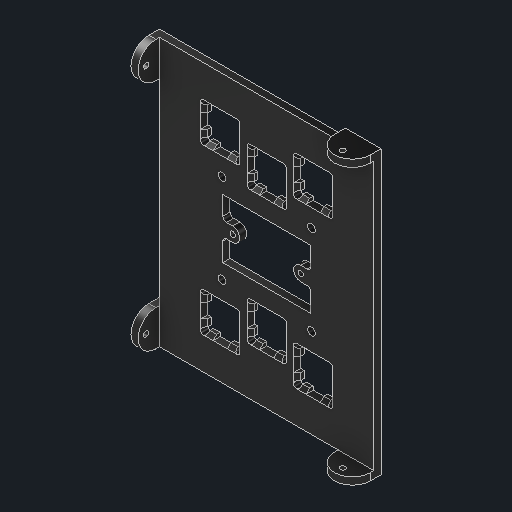
# Autodesk Inventor part: LED_mount
Saved by Autodesk Inventor 2026.1 (Build 301233000, 233)
## iProperties
Created: 2026-01-20
Part Number: LED_mount
Material: ABS Plastic
Document SubType Name: Modeling
Designer: aleja
Density: 1.06 g/cm^3
Appearance: Glossy - Black
Author: aleja
Autodesk Inventor part; units mm, degrees
ref_plane "YZ Plane" through (0, 0, 0) normal (1, 0, 0) x (0, 1, 0)
ref_plane "XZ Plane" through (0, 0, 0) normal (0, 1, 0) x (-1, 0, 0)
ref_plane "XY Plane" through (0, 0, 0) normal (0, 0, 1) x (1, 0, 0)
sketch "Sketch1" plane through (0, 0, 0) normal (0, 1, 0) x (-1, 0, 0)
  line L0 (-60, 75) -> (60, 75)
  line L1 (60, 75) -> (60, -75)
  line L2 (60, -75) -> (-60, -75)
  line L3 (-60, -75) -> (-60, 75)
  line L4 (-60, 75) -> (60, -75) construction
  line L5 (60, 75) -> (-60, -75) construction
  point P0 (0, 0)
  dimension "d0" = 120
  dimension "d1" = 150
  constraints: 12 end point, 2 midpoint, 2 parallel, 1 horizontal, 1 perpendicular
  measures "d0" distance of L1.end L2.end
  measures "d1" distance of L0.end L1.end
extrude "Extrusion1" add sketch "Sketch1" along normal blind 4
sketch "Sketch3" plane through (0, 0, 0) normal (0, -1, 0) x (1, 0, 0)
  line L0 (-60, 75) -> (60, 75) projected
  line L1 (-60, 75) -> (-64, 75)
  line L2 (-64, 75) -> (-64, 55)
  line L3 (-64, 55) -> (-60, 55)
  line L4 (-60, 55) -> (-60, 75)
  line L5 (-64, 75) -> (-40, 75)
  line L6 (-40, 75) -> (-40, 79)
  line L7 (-40, 79) -> (-64, 79)
  line L8 (-64, 79) -> (-64, 75)
  line L9 (-60, -75) -> (-60, 75) projected
  line L10 (-60, 0) -> (-43.5069, 0) construction
  line L11 (-60, -75) -> (-64, -75)
  line L12 (-64, -75) -> (-64, -55)
  line L13 (-64, -55) -> (-60, -55)
  line L14 (-60, -55) -> (-60, -75)
  line L15 (-64, -75) -> (-40, -75)
  line L16 (-40, -75) -> (-40, -79)
  line L17 (-40, -79) -> (-64, -79)
  line L18 (-64, -79) -> (-64, -75)
  line L19 (0, 75) -> (0, 63.1817) construction
  line L20 (60, 75) -> (64, 75)
  line L21 (64, 75) -> (64, 55)
  line L22 (64, 55) -> (60, 55)
  line L23 (60, 55) -> (60, 75)
  line L24 (64, 75) -> (40, 75)
  line L25 (40, 75) -> (40, 79)
  line L26 (40, 79) -> (64, 79)
  line L27 (64, 79) -> (64, 75)
  line L28 (60, -75) -> (60, 75)
  line L29 (60, 0) -> (43.5069, 0) construction
  line L30 (60, -75) -> (64, -75)
  line L31 (64, -75) -> (64, -55)
  line L32 (64, -55) -> (60, -55)
  line L33 (60, -55) -> (60, -75)
  line L34 (64, -75) -> (40, -75)
  line L35 (40, -75) -> (40, -79)
  line L36 (40, -79) -> (64, -79)
  line L37 (64, -79) -> (64, -75)
  line L38 (60, -75) -> (60, -79)
  line L39 (60, 75) -> (60, 79)
  point P0 (0, 0)
  dimension "d21" = 4
  dimension "d22" = 20
  dimension "d23" = 24
  dimension "d24" = 4
  constraints: 76 end point, 21 symmetric about line, 4 parallel, 3 horizontal, 3 perpendicular, 3 point on line, 2 midpoint, 1 vertical
  measures "d21" distance of L3.end L2.end
  measures "d22" distance of L2.end L1.end
  measures "d23" distance of L7.end L6.end
  measures "d24" distance of L6.end L5.end
extrude "Extrusion3" add sketch "Sketch3" along normal blind 15 and the other way blind 4 contours L4 L3 L2 L1 | L25 L26 L39 L0 | L11 L12 L13 L9 | L38 L36 L35 L34
sketch "Sketch2" plane through (0, 0, 0) normal (0, 1, 0) x (1, 0, 0)
  line L0 (24.55, -16.5) -> (-24.55, -16.5)
  line L1 (-24.55, -16.5) -> (-24.55, 16.5)
  line L2 (-24.55, 16.5) -> (24.55, 16.5)
  line L3 (24.55, 16.5) -> (24.55, -16.5)
  line L4 (24.55, -16.5) -> (-24.55, 16.5) construction
  line L5 (-24.55, -16.5) -> (24.55, 16.5) construction
  line L6 (-24.55, 0) -> (-19.05, 0) construction
  line L7 (0, 0) -> (0, 7.7901) construction
  line L8 (37, -57) -> (15, -57) construction
  line L9 (15, -57) -> (15, -35) construction
  line L10 (15, -35) -> (37, -35) construction
  line L11 (37, -35) -> (37, -57) construction
  line L12 (0, 0) -> (-54.7536, 0) construction
  line L13 (0, 0) -> (0, -64.3839) construction
  line L14 (-24.55, -4) -> (-19.05, -4)
  arc A0 (-19.05, -4) -> (-19.05, 4) centre (-19.05, 0) ccw
  line L15 (-24.55, 4) -> (-19.05, 4)
  circle A1 centre (-19.05, 0) radius 1.5
  line L16 (24.55, -4) -> (19.05, -4)
  arc A2 (19.05, 4) -> (19.05, -4) centre (19.05, 0) ccw
  line L17 (24.55, 4) -> (19.05, 4)
  circle A3 centre (19.05, 0) radius 1.5
  line L18 (35.4, -36.6) -> (16.6, -36.6) construction
  line L19 (16.6, -36.6) -> (16.6, -55.4) construction
  line L20 (16.6, -55.4) -> (35.4, -55.4) construction
  line L21 (35.4, -55.4) -> (35.4, -36.6) construction
  arc A4 (35, -38.1492) -> (33.8508, -37) centre (35.4, -36.6) ccw
  line L22 (26, -36.6) -> (26, -55.4) construction
  line L23 (35.4, -46) -> (16.6, -46) construction
  arc A5 (18.1492, -37) -> (17, -38.1492) centre (16.6, -36.6) ccw
  arc A6 (33.8508, -55) -> (35, -53.8508) centre (35.4, -55.4) ccw
  arc A7 (17, -53.8508) -> (18.1492, -55) centre (16.6, -55.4) ccw
  line L24 (33.8508, -37) -> (18.1492, -37)
  line L25 (33.8508, -55) -> (18.1492, -55)
  line L26 (35.4, -36.6) -> (16.6, -55.4) construction
  line L27 (16.6, -36.6) -> (35.4, -55.4) construction
  line L28 (17, -53.8508) -> (17, -38.1492)
  line L29 (35, -53.8508) -> (35, -38.1492)
  line L30 (11, -48.5) -> (-11, -48.5) construction
  line L31 (-11, -48.5) -> (-11, -26.5) construction
  line L32 (-11, -26.5) -> (11, -26.5) construction
  line L33 (11, -26.5) -> (11, -48.5) construction
  line L34 (9.4, -28.1) -> (-9.4, -28.1) construction
  line L35 (-9.4, -28.1) -> (-9.4, -46.9) construction
  line L36 (-9.4, -46.9) -> (9.4, -46.9) construction
  line L37 (9.4, -46.9) -> (9.4, -28.1) construction
  arc A8 (9, -29.6492) -> (7.8508, -28.5) centre (9.4, -28.1) ccw
  line L38 (0, -28.1) -> (0, -46.9) construction
  line L39 (9.4, -37.5) -> (-9.4, -37.5) construction
  arc A9 (-7.8508, -28.5) -> (-9, -29.6492) centre (-9.4, -28.1) ccw
  arc A10 (7.8508, -46.5) -> (9, -45.3508) centre (9.4, -46.9) ccw
  arc A11 (-9, -45.3508) -> (-7.8508, -46.5) centre (-9.4, -46.9) ccw
  line L40 (7.8508, -28.5) -> (-7.8508, -28.5)
  line L41 (7.8508, -46.5) -> (-7.8508, -46.5)
  line L42 (9.4, -28.1) -> (-9.4, -46.9) construction
  line L43 (-9.4, -28.1) -> (9.4, -46.9) construction
  line L44 (-9, -45.3508) -> (-9, -29.6492)
  line L45 (9, -45.3508) -> (9, -29.6492)
  line L46 (-37, -57) -> (-15, -57) construction
  line L47 (-15, -57) -> (-15, -35) construction
  line L48 (-15, -35) -> (-37, -35) construction
  line L49 (-37, -35) -> (-37, -57) construction
  line L50 (-35.4, -36.6) -> (-16.6, -36.6) construction
  line L51 (-16.6, -36.6) -> (-16.6, -55.4) construction
  line L52 (-16.6, -55.4) -> (-35.4, -55.4) construction
  line L53 (-35.4, -55.4) -> (-35.4, -36.6) construction
  arc A12 (-33.8508, -37) -> (-35, -38.1492) centre (-35.4, -36.6) ccw
  line L54 (-26, -36.6) -> (-26, -55.4) construction
  line L55 (-35.4, -46) -> (-16.6, -46) construction
  arc A13 (-17, -38.1492) -> (-18.1492, -37) centre (-16.6, -36.6) ccw
  arc A14 (-35, -53.8508) -> (-33.8508, -55) centre (-35.4, -55.4) ccw
  arc A15 (-18.1492, -55) -> (-17, -53.8508) centre (-16.6, -55.4) ccw
  line L56 (-33.8508, -37) -> (-18.1492, -37)
  line L57 (-33.8508, -55) -> (-18.1492, -55)
  line L58 (-35.4, -36.6) -> (-16.6, -55.4) construction
  line L59 (-16.6, -36.6) -> (-35.4, -55.4) construction
  line L60 (-17, -53.8508) -> (-17, -38.1492)
  line L61 (-35, -53.8508) -> (-35, -38.1492)
  line L62 (37, 57) -> (15, 57) construction
  line L63 (15, 57) -> (15, 35) construction
  line L64 (15, 35) -> (37, 35) construction
  line L65 (37, 35) -> (37, 57) construction
  line L66 (0, 0) -> (0, 64.3839) construction
  line L67 (35.4, 36.6) -> (16.6, 36.6) construction
  line L68 (16.6, 36.6) -> (16.6, 55.4) construction
  line L69 (16.6, 55.4) -> (35.4, 55.4) construction
  line L70 (35.4, 55.4) -> (35.4, 36.6) construction
  arc A16 (33.8508, 37) -> (35, 38.1492) centre (35.4, 36.6) ccw
  line L71 (26, 36.6) -> (26, 55.4) construction
  line L72 (35.4, 46) -> (16.6, 46) construction
  arc A17 (17, 38.1492) -> (18.1492, 37) centre (16.6, 36.6) ccw
  arc A18 (35, 53.8508) -> (33.8508, 55) centre (35.4, 55.4) ccw
  arc A19 (18.1492, 55) -> (17, 53.8508) centre (16.6, 55.4) ccw
  line L73 (33.8508, 37) -> (18.1492, 37)
  line L74 (33.8508, 55) -> (18.1492, 55)
  line L75 (35.4, 36.6) -> (16.6, 55.4) construction
  line L76 (16.6, 36.6) -> (35.4, 55.4) construction
  line L77 (17, 53.8508) -> (17, 38.1492)
  line L78 (35, 53.8508) -> (35, 38.1492)
  arc A20 (7.8508, 28.5) -> (9, 29.6492) centre (9.4, 28.1) ccw
  line L79 (9, 45.3508) -> (9, 29.6492)
  line L80 (9.4, 46.9) -> (9.4, 28.1) construction
  line L81 (11, 26.5) -> (11, 48.5) construction
  arc A21 (9, 45.3508) -> (7.8508, 46.5) centre (9.4, 46.9) ccw
  line L82 (7.8508, 28.5) -> (-7.8508, 28.5)
  line L83 (-11, 26.5) -> (11, 26.5) construction
  line L84 (0, 28.1) -> (0, 46.9) construction
  line L85 (9.4, 28.1) -> (-9.4, 28.1) construction
  line L86 (9.4, 37.5) -> (-9.4, 37.5) construction
  line L87 (-9, 45.3508) -> (-9, 29.6492)
  line L88 (-9.4, 28.1) -> (9.4, 46.9) construction
  line L89 (9.4, 28.1) -> (-9.4, 46.9) construction
  line L90 (-9.4, 28.1) -> (-9.4, 46.9) construction
  line L91 (7.8508, 46.5) -> (-7.8508, 46.5)
  line L92 (-9.4, 46.9) -> (9.4, 46.9) construction
  line L93 (11, 48.5) -> (-11, 48.5) construction
  line L94 (-11, 48.5) -> (-11, 26.5) construction
  arc A22 (-9, 29.6492) -> (-7.8508, 28.5) centre (-9.4, 28.1) ccw
  arc A23 (-7.8508, 46.5) -> (-9, 45.3508) centre (-9.4, 46.9) ccw
  line L95 (-37, 57) -> (-15, 57) construction
  line L96 (-15, 57) -> (-15, 35) construction
  line L97 (-33.8508, 55) -> (-18.1492, 55)
  line L98 (-16.6, 36.6) -> (-35.4, 55.4) construction
  line L99 (-35.4, 36.6) -> (-16.6, 55.4) construction
  arc A24 (-17, 53.8508) -> (-18.1492, 55) centre (-16.6, 55.4) ccw
  line L100 (-16.6, 55.4) -> (-35.4, 55.4) construction
  line L101 (-16.6, 36.6) -> (-16.6, 55.4) construction
  line L102 (-17, 53.8508) -> (-17, 38.1492)
  line L103 (-35.4, 46) -> (-16.6, 46) construction
  line L104 (-33.8508, 37) -> (-18.1492, 37)
  line L105 (-35.4, 36.6) -> (-16.6, 36.6) construction
  arc A25 (-18.1492, 37) -> (-17, 38.1492) centre (-16.6, 36.6) ccw
  line L106 (-15, 35) -> (-37, 35) construction
  arc A26 (-35, 38.1492) -> (-33.8508, 37) centre (-35.4, 36.6) ccw
  line L107 (-26, 36.6) -> (-26, 55.4) construction
  line L108 (-35, 53.8508) -> (-35, 38.1492)
  line L109 (-37, 35) -> (-37, 57) construction
  arc A27 (-33.8508, 55) -> (-35, 53.8508) centre (-35.4, 55.4) ccw
  line L110 (-35.4, 55.4) -> (-35.4, 36.6) construction
  point P0 (19.05, 0)
  dimension "d4" = 49.1
  dimension "d5" = 33
  dimension "d64" = 22
  dimension "d66" = 15
  dimension "d68" = 35
  dimension "d82" = 5.5
  dimension "d83" = 3
  dimension "d85" = 8
  dimension "d119" = 18.8
  dimension "d120" = 3.2
  dimension "d121" = 2
  dimension "d122" = 22
  dimension "d123" = 18.8
  dimension "d124" = 3.2
  dimension "d125" = 2
  dimension "d126" = 10
  constraints: 222 end point, 122 symmetric about line, 52 point on circle, 28 centre point, 11 midpoint, 10 parallel, 9 horizontal, 8 coincident, 7 perpendicular, 4 tangent, 3 point on line, 2 vertical, 1 collinear, 30 other
  measures "d4" distance of L1.end L2.end
  measures "d5" distance of L0.end L1.end
  measures "d64" distance of L8.start L8.end
  measures "d66" distance from line of L7.start L9
  measures "d68" distance from line of L7.start L10
  measures "d82" distance of L15.end L15.start
  measures "d83" diameter of A1
  measures "d85" distance between parallel lines of L15 L14
  measures "d119" distance of L20.end L18.start
  measures "d120" diameter of A4
  measures "d121" distance between parallel lines of L10 L24
  measures "d122" distance of L33.end L30.end
  measures "d123" distance of L37.start L37.end
  measures "d124" diameter of A8
  measures "d125" distance between parallel lines of L32 L40
  measures "d126" distance between parallel lines of L0 L32
extrude "Extrusion2" cut sketch "Sketch2" along normal through all contours L0 L1 L14 A0 L15 L2 L3 L17 A2 L16 | A1 | A3 | L29 A6 L25 A7 L28 A5 L24 A4 | L45 A10 L41 A11 L44 A9 L40 A8 | L56 A13 L60 A15 L57 A14 L61 A12 | L73 A17 L77 A19 L74 A18 L78 A16 | L82 A22 L87 A23 L91 A21 L79 A20 | L97 A24 L102 A25 L104 A26 L108 A27
sketch "Sketch7" plane through (-60, 0, -55) normal (1, 0, 0) x (0, 0, -1)
  line L0 (0, -15) -> (20, -15) projected
  line L1 (10, -15) -> (10, 0)
  line L2 (20, 0) -> (0, 0) projected
  circle A0 centre (10, -7.5) radius 1.5
  line L3 (-55, 0) -> (-55, -12.3055)
  circle A1 centre (-120, -7.5) radius 1.5
  dimension "d47" = 3
  constraints: 4 end point, 3 midpoint, 2 centre point, 1 symmetric about line, 1 vertical, 1 other
  measures "d47" diameter of A0
extrude "Extrusion8" cut sketch "Sketch7" against normal through all
sketch "Sketch8" plane through (60, 0, 75) normal (0, 0, -1) x (-1, 0, 0)
  line L0 (20, -15) -> (0, -15) projected
  line L1 (10, -15) -> (10, 0)
  line L2 (20, 0) -> (0, 0) projected
  circle A0 centre (10, -7.5) radius 1.5
  point P0 (60, 0)
  dimension "d50" = 3
  constraints: 3 midpoint, 2 end point, 1 centre point
  measures "d50" diameter of A0
extrude "Extrusion9" cut sketch "Sketch8" along normal through all both and the other way through all
sketch "Sketch9" plane through (0, -15, 0) normal (0, -1, 0) x (1, 0, 0)
  line L0 (-64, -55) -> (-64, -75) projected
  line L1 (-60, -75) -> (-60, -55) projected
  line L2 (-60, -55) -> (-64, -55) projected
  line L3 (-64, -75) -> (-60, -75) projected
  line L4 (-64, 55) -> (-60, 55) projected
  line L5 (-60, 55) -> (-60, 75) projected
  line L6 (-60, 75) -> (-64, 75) projected
  line L7 (-64, 75) -> (-64, 55) projected
  line L8 (60, 79) -> (40, 79) projected
  line L9 (40, 79) -> (40, 75) projected
  line L10 (40, 75) -> (60, 75) projected
  line L11 (60, 75) -> (60, 79) projected
  line L12 (40, -79) -> (60, -79) projected
  line L13 (60, -79) -> (60, -75) projected
  line L14 (60, -75) -> (40, -75) projected
  line L15 (40, -75) -> (40, -79) projected
  point P0 (0, 0)
extrude "Extrusion10" cut sketch "Sketch9" against normal blind 3
fillet "Fillet2" radius 10 8 edges at (-62, -12, -55) (-62, -12, -75) (-62, -12, 55) (-62, -12, 75) (40, -12, 77) (60, -12, 77) (60, -12, -77) (40, -12, -77)
sketch "Sketch10" plane through (0, 4, 0) normal (0, 1, 0) x (1, 0, 0)
  line L0 (25, 25) -> (-25, 25) construction
  line L1 (-25, 25) -> (-25, -25) construction
  line L2 (-25, -25) -> (25, -25) construction
  line L3 (25, -25) -> (25, 25) construction
  line L4 (25, 25) -> (-25, -25) construction
  line L5 (-25, 25) -> (25, -25) construction
  circle A0 centre (25, -25) radius 2.15
  circle A1 centre (-25, -25) radius 2.15
  circle A2 centre (-25, 25) radius 2.15
  circle A3 centre (25, 25) radius 2.15
  point P0 (0, 0)
  dimension "d56" = 50
  dimension "d57" = 50
  dimension "d58" = 4.3
  dimension "d59" = 4.3
  dimension "d60" = 4.3
  dimension "d61" = 4.3
  constraints: 12 end point, 4 centre point, 4 coincident, 2 midpoint, 2 parallel, 1 horizontal, 1 perpendicular
  measures "d56" distance of L1.end L2.end
  measures "d57" distance of L0.end L1.end
  measures "d58" diameter of A0
  measures "d59" diameter of A1
  measures "d60" diameter of A2
  measures "d61" diameter of A3
extrude "Extrusion12" cut sketch "Sketch10" against normal through all
fillet "Fillet3" radius 2 4 edges at (-24.55, 2, -4) (-24.55, 2, 4) (24.55, 2, 4) (24.55, 2, -4)
chamfer "Chamfer2" distance 2 angle 45 24 edges at (0, 0, -46.5) (26, 0, -55) (35, 0, -46) (17, 0, -46) (26, 0, -37) (9, 0, -37.5) (0, 0, -28.5) (-9, 0, -37.5) (-17, 0, -46) (-26, 0, -55) (-26, 0, -37) (-35, 0, -46) (-26, 0, 37) (-17, 0, 46) (-26, 0, 55) (-35, 0, 46) (-9, 0, 37.5) (0, 0, 46.5) (9, 0, 37.5) (0, 0, 28.5) (26, 0, 37) (35, 0, 46) (26, 0, 55) (17, 0, 46)
sketch "Sketch14" plane through (0, 0, 0) normal (0, -1, 0) x (1, 0, 0)
  line L0 (60, -75) -> (40, -75) projected
  line L1 (60, 75) -> (60, -75) projected
  line L2 (40, 75) -> (60, 75) projected
  line L3 (-60, 75) -> (40, 75) projected
  line L4 (-60, 55) -> (-60, 75) projected
  line L5 (-60, -55) -> (-60, 55) projected
  line L6 (-60, -75) -> (-60, -55) projected
  line L7 (40, -75) -> (-60, -75) projected
  line L8 (-11, -28.1) -> (-11, -46.9) projected
  arc A0 (-9.4, -26.5) -> (-11, -28.1) centre (-9.4, -28.1) ccw projected
  line L9 (9.4, -26.5) -> (-9.4, -26.5) projected
  arc A1 (11, -28.1) -> (9.4, -26.5) centre (9.4, -28.1) ccw projected
  line L10 (11, -46.9) -> (11, -28.1) projected
  arc A2 (9.4, -48.5) -> (11, -46.9) centre (9.4, -46.9) ccw projected
  line L11 (-9.4, -48.5) -> (9.4, -48.5) projected
  arc A3 (-11, -46.9) -> (-9.4, -48.5) centre (-9.4, -46.9) ccw projected
  line L12 (-37, 55.4) -> (-37, 36.6) projected
  arc A4 (-35.4, 57) -> (-37, 55.4) centre (-35.4, 55.4) ccw projected
  line L13 (-16.6, 57) -> (-35.4, 57) projected
  arc A5 (-15, 55.4) -> (-16.6, 57) centre (-16.6, 55.4) ccw projected
  line L14 (-15, 36.6) -> (-15, 55.4) projected
  arc A6 (-16.6, 35) -> (-15, 36.6) centre (-16.6, 36.6) ccw projected
  line L15 (-35.4, 35) -> (-16.6, 35) projected
  arc A7 (-37, 36.6) -> (-35.4, 35) centre (-35.4, 36.6) ccw projected
  circle A8 centre (19.05, 0) radius 1.5 projected
  line L16 (15, 55.4) -> (15, 36.6) projected
  arc A9 (16.6, 57) -> (15, 55.4) centre (16.6, 55.4) ccw projected
  line L17 (35.4, 57) -> (16.6, 57) projected
  arc A10 (37, 55.4) -> (35.4, 57) centre (35.4, 55.4) ccw projected
  line L18 (37, 36.6) -> (37, 55.4) projected
  arc A11 (35.4, 35) -> (37, 36.6) centre (35.4, 36.6) ccw projected
  line L19 (16.6, 35) -> (35.4, 35) projected
  arc A12 (15, 36.6) -> (16.6, 35) centre (16.6, 36.6) ccw projected
  line L20 (-37, -36.6) -> (-37, -55.4) projected
  arc A13 (-35.4, -35) -> (-37, -36.6) centre (-35.4, -36.6) ccw projected
  line L21 (-16.6, -35) -> (-35.4, -35) projected
  arc A14 (-15, -36.6) -> (-16.6, -35) centre (-16.6, -36.6) ccw projected
  line L22 (-15, -55.4) -> (-15, -36.6) projected
  arc A15 (-16.6, -57) -> (-15, -55.4) centre (-16.6, -55.4) ccw projected
  line L23 (-35.4, -57) -> (-16.6, -57) projected
  arc A16 (-37, -55.4) -> (-35.4, -57) centre (-35.4, -55.4) ccw projected
  line L24 (-9.4, 26.5) -> (9.4, 26.5) projected
  arc A17 (-11, 28.1) -> (-9.4, 26.5) centre (-9.4, 28.1) ccw projected
  line L25 (-11, 46.9) -> (-11, 28.1) projected
  arc A18 (-9.4, 48.5) -> (-11, 46.9) centre (-9.4, 46.9) ccw projected
  line L26 (9.4, 48.5) -> (-9.4, 48.5) projected
  arc A19 (11, 46.9) -> (9.4, 48.5) centre (9.4, 46.9) ccw projected
  line L27 (11, 28.1) -> (11, 46.9) projected
  arc A20 (9.4, 26.5) -> (11, 28.1) centre (9.4, 28.1) ccw projected
  circle A21 centre (-19.05, 0) radius 1.5 projected
  line L28 (-24.55, 16.5) -> (24.55, 16.5) projected
  line L29 (24.55, 16.5) -> (24.55, 6) projected
  arc A22 (22.55, 4) -> (24.55, 6) centre (22.55, 6) ccw projected
  line L30 (22.55, 4) -> (19.05, 4) projected
  arc A23 (19.05, 4) -> (19.05, -4) centre (19.05, 0) ccw projected
  line L31 (19.05, -4) -> (22.55, -4) projected
  arc A24 (24.55, -6) -> (22.55, -4) centre (22.55, -6) ccw projected
  line L32 (24.55, -6) -> (24.55, -16.5) projected
  line L33 (24.55, -16.5) -> (-24.55, -16.5) projected
  line L34 (-24.55, -16.5) -> (-24.55, -6) projected
  arc A25 (-22.55, -4) -> (-24.55, -6) centre (-22.55, -6) ccw projected
  line L35 (-22.55, -4) -> (-19.05, -4) projected
  arc A26 (-19.05, -4) -> (-19.05, 4) centre (-19.05, 0) ccw projected
  line L36 (-19.05, 4) -> (-22.55, 4) projected
  arc A27 (-24.55, 6) -> (-22.55, 4) centre (-22.55, 6) ccw projected
  line L37 (-24.55, 6) -> (-24.55, 16.5) projected
  circle A28 centre (25, 25) radius 2.15 projected
  circle A29 centre (25, -25) radius 2.15 projected
  circle A30 centre (-25, 25) radius 2.15 projected
  circle A31 centre (-25, -25) radius 2.15 projected
  line L38 (35.4, -35) -> (16.6, -35) projected
  arc A32 (37, -36.6) -> (35.4, -35) centre (35.4, -36.6) ccw projected
  line L39 (37, -55.4) -> (37, -36.6) projected
  arc A33 (35.4, -57) -> (37, -55.4) centre (35.4, -55.4) ccw projected
  line L40 (16.6, -57) -> (35.4, -57) projected
  arc A34 (15, -55.4) -> (16.6, -57) centre (16.6, -55.4) ccw projected
  line L41 (15, -36.6) -> (15, -55.4) projected
  arc A35 (16.6, -35) -> (15, -36.6) centre (16.6, -36.6) ccw projected
  line L42 (37, 50) -> (15, 50)
  line L43 (15, 50) -> (15, 42)
  line L44 (15, 42) -> (37, 42)
  line L45 (37, 42) -> (37, 50)
  line L46 (37, 36.6) -> (37, 55.4) projected
  line L47 (30, 57) -> (22, 57)
  line L48 (22, 57) -> (22, 35)
  line L49 (22, 35) -> (30, 35)
  line L50 (30, 35) -> (30, 57)
  line L51 (35.4, 57) -> (16.6, 57) projected
  line L52 (11, 28.1) -> (11, 46.9) projected
  line L53 (11, 41.5) -> (-11, 41.5)
  line L54 (-11, 41.5) -> (-11, 33.5)
  line L55 (-11, 33.5) -> (11, 33.5)
  line L56 (11, 33.5) -> (11, 41.5)
  line L57 (-11, 46.9) -> (-11, 28.1) projected
  line L58 (4, 48.5) -> (-4, 48.5)
  line L59 (-4, 48.5) -> (-4, 26.5)
  line L60 (-4, 26.5) -> (4, 26.5)
  line L61 (4, 26.5) -> (4, 48.5)
  line L62 (9.4, 48.5) -> (-9.4, 48.5) projected
  line L63 (0, 0) -> (0, -8.3833) construction
  line L64 (-15, 55.4) -> (-15, 36.6)
  arc A36 (-15, 55.4) -> (-16.6, 57) centre (-16.6, 55.4) ccw
  line L65 (-35.4, 57) -> (-16.6, 57)
  arc A37 (-35.4, 57) -> (-37, 55.4) centre (-35.4, 55.4) ccw
  line L66 (-37, 36.6) -> (-37, 55.4)
  arc A38 (-37, 36.6) -> (-35.4, 35) centre (-35.4, 36.6) ccw
  line L67 (-16.6, 35) -> (-35.4, 35)
  arc A39 (-16.6, 35) -> (-15, 36.6) centre (-16.6, 36.6) ccw
  line L68 (-37, 50) -> (-15, 50)
  line L69 (-15, 50) -> (-15, 42)
  line L70 (-15, 42) -> (-37, 42)
  line L71 (-37, 42) -> (-37, 50)
  line L72 (-37, 36.6) -> (-37, 55.4)
  line L73 (-30, 57) -> (-22, 57)
  line L74 (-22, 57) -> (-22, 35)
  line L75 (-22, 35) -> (-30, 35)
  line L76 (-30, 35) -> (-30, 57)
  line L77 (-35.4, 57) -> (-16.6, 57)
  line L78 (0, 0) -> (-11, 0) construction
  line L79 (37, -50) -> (15, -50)
  line L80 (15, -42) -> (37, -42)
  line L81 (22, -57) -> (22, -35)
  line L82 (30, -35) -> (30, -57)
  line L83 (11, -41.5) -> (-11, -41.5)
  line L84 (-11, -33.5) -> (11, -33.5)
  line L85 (-4, -48.5) -> (-4, -26.5)
  line L86 (4, -26.5) -> (4, -48.5)
  line L87 (-30, -35) -> (-30, -57)
  line L88 (-15, -42) -> (-37, -42)
  line L89 (-37, -50) -> (-15, -50)
  line L90 (-22, -57) -> (-22, -35)
  point P0 (37, 46)
  point P1 (37, 46)
  point P2 (26, 57)
  point P3 (26, 57)
  point P4 (-11, 37.5)
  point P5 (-11, 37.5)
  point P6 (0, 48.5)
  point P7 (0, 48.5)
  point P8 (-37, 46)
  point P9 (-37, 46)
  point P10 (-26, 57)
  point P11 (-26, 57)
  point P12 (22, -42)
  point P13 (15, -50)
  point P14 (22, -50)
  point P15 (30, -50)
  point P16 (30, -42)
  point P17 (-22, -42)
  point P18 (-30, -42)
  point P19 (-30, -50)
  point P20 (-22, -50)
  point P21 (-15, -50)
  point P22 (-22, 42)
  point P23 (-15, 50)
  point P24 (-22, 50)
  point P25 (-30, 50)
  point P26 (-30, 42)
  point P27 (4, 41.5)
  point P28 (4, 33.5)
  point P29 (-4, 33.5)
  point P30 (-4, 41.5)
  point P31 (-11, 41.5)
  point P32 (30, 50)
  point P33 (30, 42)
  point P34 (22, 42)
  point P35 (22, 50)
  point P36 (15, 50)
  point P37 (-4, -41.5)
  point P38 (4, -41.5)
  point P39 (4, -33.5)
  point P40 (-4, -33.5)
  point P41 (-11, -41.5)
  dimension "d133" = 4
  dimension "d134" = 4
  dimension "d135" = 4
  dimension "d136" = 4
  dimension "d137" = 4
  dimension "d138" = 4
  dimension "d139" = 4
  dimension "d140" = 4
  constraints: 88 end point, 40 symmetric about line, 12 point on line, 8 midpoint, 8 parallel, 8 point on circle, 5 horizontal, 4 centre point, 4 perpendicular, 1 vertical, 4 other
  measures "d133" distance from line of L44 point (37, 46)
  measures "d134" distance from line of point (37, 46) L42
  measures "d135" distance from line of point (26, 57) L50
  measures "d136" distance from line of point (26, 57) L48
  measures "d137" distance from line of point (-11, 37.5) L55
  measures "d138" distance from line of point (-11, 37.5) L53
  measures "d139" distance from line of point (0, 48.5) L61
  measures "d140" distance from line of L59 point (0, 48.5)
extrude "Extrusion15" cut sketch "Sketch14" against normal through all contours L84 L85 L83 L8 | L85 L9 L86 L84 | L84 L86 L83 L85 | L83 L86 L11 L85 | L84 L10 L83 L86 | L68 L76 L70 L12 | L76 L13 L74 L68 | L68 L74 L70 L76 | L70 L74 L15 L76 | L68 L14 L70 L74 | L42 L48 L44 L16 | L48 L17 L50 L42 | L44 L50 L19 L48 | L42 L18 L44 L50 | L88 L87 L89 L20 | L88 L90 L89 L87 | L87 L21 L90 L88 | L89 L90 L23 L87 | L88 L22 L89 L90 | L59 L55 L61 L24 | L55 L25 L53 L59 | L61 L53 L27 L55 | L59 L26 L61 L53 | L82 L80 L81 L38 | L82 L79 L81 L80 | L80 L39 L79 L82 | L81 L79 L41 L80 | L82 L40 L81 L79
body "Solid1"
